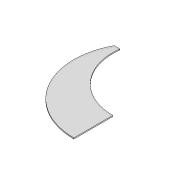
# Autodesk Inventor part: Part1
Saved by Autodesk Inventor 2022 (Build 260153000, 153)
## iProperties
Created: 2022-04-29
Part Number: Part1
Material: Generic
Document SubType Name: Modeling
Designer: alber
Density: 1 g/cm^3
Appearance: Default
Author: alber
Autodesk Inventor part; units mm, degrees
ref_plane "YZ Plane" through (0, 0, 0) normal (1, 0, 0) x (0, 1, 0)
ref_plane "XZ Plane" through (0, 0, 0) normal (0, 1, 0) x (-1, 0, 0)
ref_plane "XY Plane" through (0, 0, 0) normal (0, 0, 1) x (1, 0, 0)
sketch "Sketch1" plane through (0, 0, 0) normal (0, 1, 0) x (-1, 0, 0)
  arc A0 (53.6656, -29) -> (0, 61) centre (0, 0) ccw
  arc A1 (48.6313, -29) -> (0, 26) centre (0, -23) ccw
  line L0 (53.6656, -29) -> (48.6313, -29)
  line L1 (0, 61) -> (0, 26)
  line L2 (0, -50.0482) -> (0, 97.2892) projected
  arc A2 (49.6387, -29) -> (0, 27) centre (0, -23) ccw
  arc A3 (52.5262, -29) -> (0, 60) centre (0, 0) ccw
  dimension "d3" = 90
  dimension "d6" = 35
  dimension "d7" = 49
  dimension "d8" = 61
  dimension "d10" = 60
  dimension "d11" = 50
  dimension "d12" = 23
  constraints: 8 point on circle, 5 point on line, 4 centre point, 4 end point, 3 coincident, 1 collinear, 1 horizontal, 1 vertical
  measures "d3" vertical distance of L0.end L1.start
  measures "d6" distance of L1.start L1.end
  measures "d7" radius of A1
  measures "d8" radius of A0
  measures "d10" radius of A3
  measures "d11" radius of A2
  measures "d12" distance of A1.centre point (0, 0)
extrude "Extrusion1" add sketch "Sketch1" along normal blind 1
body "Solid1"
